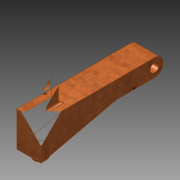
# Autodesk Inventor part: Swinging_connection
Saved by Autodesk Inventor 2015 (Build 190159000, 159)
## iProperties
Created: 2017-02-21
Part Number: Swinging_connection
Material: Wood (Cherry)
Document SubType Name: Modeling
Designer: Guy
Density: 0.63 g/cm^3
Appearance: Cherry - Natural Low Gloss
Author: Guy
Autodesk Inventor part; units mm, degrees
ref_plane "YZ Plane" through (0, 0, 0) normal (1, 0, 0) x (0, 1, 0)
ref_plane "XZ Plane" through (0, 0, 0) normal (0, 1, 0) x (-1, 0, 0)
ref_plane "XY Plane" through (0, 0, 0) normal (0, 0, 1) x (1, 0, 0)
sketch "Sketch1" plane through (0, 0, 0) normal (0, 0, 1) x (1, 0, 0)
  line L0 (0, 0) -> (-70, 0)
  line L1 (0, 0) -> (0, -10)
  line L2 (0, -10) -> (-26.6667, -10)
  line L3 (-26.6667, -10) -> (-70, -20)
  line L4 (-70, -20) -> (-70, 0)
  circle A0 centre (-5, -5) radius 2.5
  dimension "d0" = 70
  dimension "d1" = 5
  dimension "d2" = 10
  dimension "d3" = 5
  dimension "d4" = 5
  dimension "d5" = 20
  constraints: 10 end point, 2 horizontal, 1 centre point, 1 perpendicular, 1 point on line, 1 vertical
  measures "d0" distance of L0.start L0.end
  measures "d1" diameter of A0
  measures "d2" distance between parallel lines of L2 L0
  measures "d3" distance from line of A0.centre L0
  measures "d4" distance from line of A0.centre L1
  measures "d5" distance of L3.end L0.end
extrude "Extrusion1" add sketch "Sketch1" along normal blind 14
sketch "Sketch2" plane through (-70, 0, 0) normal (0, 1, 0) x (1, 0, 0)
  line L0 (15, -5) -> (0, -5)
  line L1 (0, -5) -> (0, -9)
  line L2 (0, -9) -> (15, -9)
  line L3 (15, -9) -> (15, -5)
  line L4 (70, -14) -> (0, -14) projected
  line L5 (70, 0) -> (0, 0) projected
  line L6 (0, 0) -> (0, -14) projected
  line L7 (70, -14) -> (0, -14) projected
  line L8 (70, 0) -> (70, -14) projected
  line L9 (0, 0) -> (0, -14) projected
  dimension "d8" = 4
  dimension "d9" = 5
  dimension "d10" = 15
  constraints: 8 end point, 2 parallel, 1 horizontal, 1 perpendicular, 1 point on line
  measures "d8" distance of L2.end L0.start
  measures "d9" distance between parallel lines of L4 L2
  measures "d10" distance of L0.start L0.end
extrude "Extrusion2" add sketch "Sketch2" along normal blind 15 contours L3 L2 L1 L0
sketch "Sketch3" plane through (-70, 0, 9) normal (0, 0, 1) x (1, 0, 0)
  line L0 (15, 0) -> (0, 0) projected
  line L1 (15, 0) -> (15, 15) projected
  line L2 (0, 15) -> (15, 15) projected
  line L3 (0, 0) -> (0, 15) projected
  circle A0 centre (10, 10) radius 3
  point P0 (70, 0)
  dimension "d14" = 6
  dimension "d15" = 5
  dimension "d16" = 5
  constraints: 1 centre point
  measures "d14" diameter of A0
  measures "d15" distance from line of L1 A0.centre
  measures "d16" distance from line of A0.centre L2
extrude "Extrusion3" cut sketch "Sketch3" against normal blind 8 contours A0
fillet "Fillet3" radius 3 2 edges at (-70, 15, 7) (-55, 15, 7)
fillet "Fillet4" radius 4 1 edges at (-26.6667, -10, 7)
fillet "Fillet5" radius 5 2 edges at (0, 0, 7) (0, -10, 7)
sketch "Sketch4" plane through (-70, -20, 0) normal (0.2248595, -0.9743912, 0) x (0.9743912, 0.2248595, 0)
  circle A0 centre (6, 7) radius 4
  line L0 (44.0167, 14) -> (44.0167, 0) projected
  line L1 (0, 14) -> (44.0167, 14) projected
  line L2 (0, 0) -> (0, 14) projected
  line L3 (0, 0) -> (44.0167, 0) projected
  point P0 (72.7046, 0)
  dimension "d24" = 8
  dimension "d25" = 6
  dimension "d26" = 7
  constraints: 1 centre point
  measures "d24" diameter of A0
  measures "d25" distance from line of L2 A0.centre
  measures "d26" distance from line of L1 A0.centre
extrude "Extrusion4" add sketch "Sketch4" along normal blind 5 contours A0
fillet "Fillet6" radius 1 1 edges at (-66.9269, -24.4222, 7)
fillet "Fillet7" radius 1.5 3 edges at (-62.5, 0, 9) (-62.5, 0, 5) (-55, 0, 7)
body "Solid1"
